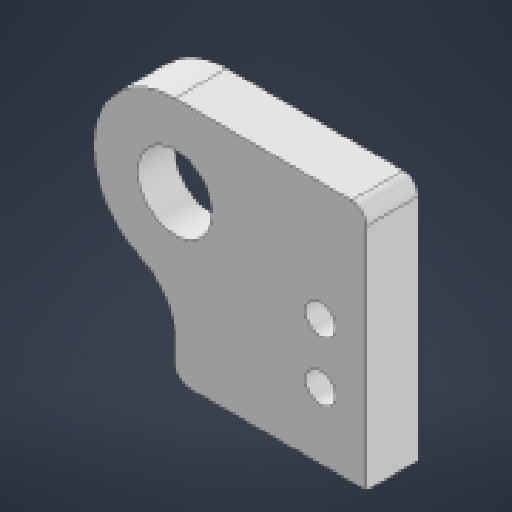
# Autodesk Inventor part: 针头装配体
Saved by Autodesk Inventor 2025 (Build 290162000, 162)
## iProperties
Created: 2025-12-07
Part Number: 针头装配体
Material: 常规
Document SubType Name: Modeling
Designer: XH
Density: 1 g/cm^3
Appearance: 默认
Author: XH
Autodesk Inventor part; units mm, degrees
ref_plane "YZ Plane" through (0, 0, 0) normal (1, 0, 0) x (0, 1, 0)
ref_plane "XZ Plane" through (0, 0, 0) normal (0, 1, 0) x (-1, 0, 0)
ref_plane "XY Plane" through (0, 0, 0) normal (0, 0, 1) x (1, 0, 0)
sketch "草图1" plane through (0, 0, 0) normal (0, 0, 1) x (1, 0, 0)
  circle A0 centre (-1.9411, 0.0503) radius 2.5
  line L0 (4.3454, -10.9196) -> (9.6453, -10.9355) projected
  circle A1 centre (-1.9411, 0.0503) radius 5.5
  line L1 (-1.9411, -10.9276) -> (10.9921, -10.9276)
  line L2 (10.9921, -10.9276) -> (10.9921, 5.5503)
  line L3 (10.9921, 5.5503) -> (-1.9411, 5.5503)
  line L4 (-1.9411, 5.5503) -> (-1.9411, -10.9276)
  point P0 (6.9953, -10.9276)
  point P1 (-1.9411, 5.5503)
  point P2 (-1.9411, -5.4497)
  dimension "d3" = 3
  dimension "d5" = 5
  constraints: 8 end point, 2 parallel, 2 point on line, 1 centre point, 1 coincident, 1 horizontal, 1 midpoint, 1 perpendicular, 3 other
  measures "d5" diameter of A0
extrude "拉伸1" add sketch "草图1" along normal blind 3.5 contours A0 L4 A1 | A0 L4 A1 | L3 L2 L1 L4 A1
fillet "圆角1" radius 4 1 edges at (-1.9411, -5.4497, 1.75)
sketch "草图2" plane through (0, 0, 0) normal (0, 0, -1) x (-1, 0, 0)
  point P0 (0, 0)
sketch "草图3" plane through (0, 0, 0) normal (0, 0, -1) x (-1, 0, 0)
  circle A0 centre (1.9411, 0.0503) radius 2.5 projected
  circle A1 centre (1.9411, 0.0503) radius 4
  point P0 (0, 0)
  dimension "d6" = 8
  constraints: 1 centre point, 1 coincident
  measures "d6" diameter of A1
extrude "拉伸2" cut sketch "草图3" against normal blind 1 contours A0 | A1
sketch "草图4" plane through (-1.9411, -10.9276, 0) normal (0, -1, 0) x (1, 0, 0)
  ellipse E0 centre (8.9346, 1.75) end of major axis (8.9346, 0.85) minor radius 0.9 projected
  point P0 (1.9411, 0)
extrude "拉伸3" cut sketch "草图4" against normal blind 3
fillet "圆角2" radius 1 2 edges at (10.9921, 5.5503, 1.75) (-1.9411, -10.9276, 1.75)
sketch "草图5" plane through (0, 0, 3.5) normal (0, 0, 1) x (1, 0, 0)
  line L0 (15.1126, -4.4497) -> (15.1126, -8.4497) projected
  line L1 (5.3617, -4.4497) -> (15.1126, -4.4497) projected
  line L2 (5.3617, -8.4497) -> (5.3617, -4.4497) projected
  line L3 (5.3617, -8.4497) -> (15.1126, -8.4497) projected
  line L4 (5.3617, -6.4497) -> (10.3955, -6.4497)
  circle A0 centre (7.8786, -6.4497) radius 1
  circle A1 centre (7.8786, -6.4497) radius 1 projected
  point P0 (0, 0)
  dimension "d12" = 2
  constraints: 2 end point, 2 midpoint, 1 centre point, 1 horizontal
  measures "d12" diameter of A0
extrude "拉伸4" cut sketch "草图5" against normal blind 5.5 contours A0 L4 | L4 A0
sketch "草图6" plane through (0, 0, 3.5) normal (0, 0, 1) x (1, 0, 0)
  circle A0 centre (7.8786, -2.4497) radius 1 projected
  point P0 (0, 0)
extrude "拉伸5" cut sketch "草图6" against normal blind 10
